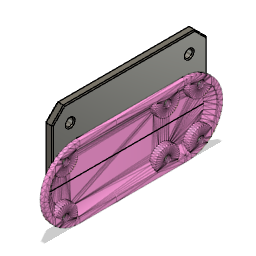
btt-smart-filament-sensor-mount (Autodesk Fusion 360 design; units mm, degrees)
Autodesk Fusion 360 part; units mm, degrees
note: some values were not read from the file. Set by a fixed rule: which sketch regions a step uses.
other "Base Mesh Feature1"
other "Modify1"
sketch "Sketch1" plane through (0, 0, 0) normal (1, 0, 0) x (0, 0, -1)
  line L0 (-32.5, 0) -> (32.5, 0)
  line L1 (32.5, 0) -> (32.5, 24.5)
  line L2 (27.5, 29.5) -> (-27.5, 29.5)
  line L3 (-32.5, 24.5) -> (-32.5, 0)
  line L4 (0, 29.5) -> (0, 0) construction
  circle A0 centre (-25, 22) radius 1.625
  circle A1 centre (25, 22) radius 1.625
  line L5 (27.5, 29.5) -> (32.5, 24.5)
  line L6 (-32.5, 24.5) -> (-27.5, 29.5)
  circle A2 centre (-28.3961, 10.1888) radius 1.5
  circle A3 centre (14.3954, 10.181) radius 1.5
  circle A4 centre (28.3567, 10.1798) radius 1.5
  circle A5 centre (28.3567, 10.1798) radius 3
  circle A6 centre (14.3954, 10.181) radius 3
  circle A7 centre (-28.3961, 10.1888) radius 3
  circle A8 centre (-28.3961, -10.2259) radius 3
  circle A9 centre (14.3954, -10.167) radius 3
  circle A10 centre (28.4406, -10.167) radius 3
  line L7 (22.5, 13) -> (-22.5, 13)
  arc A11 (32.5, 8.2913) -> (22.5, 13) centre (22.5, 0.027) ccw
  line L8 (32.5, 11.1601) -> (31.2931, 9.5653) construction
  arc A12 (-22.5, 13) -> (-32.5, 8.292) centre (-22.5, 0.0257) ccw
  line L9 (-32.5, 11.1715) -> (-31.1644, 9.6829) construction
  line L10 (-31.1644, 9.6829) -> (-32.653, 8.3472) construction
  line L11 (31.2931, 9.5653) -> (32.8879, 8.3584) construction
  point P0 (32.5, 11.1601)
  point P1 (-32.5, 11.1715)
  dimension "d1" = 3.25
  dimension "d2" = 25
  dimension "d3" = 22
  dimension "d4" = 5
  dimension "d5" = 5
  dimension "d6" = 5
  dimension "d7" = 5
  dimension "d8" = 7.5
  dimension "d13" = 3
  dimension "d14" = 3
  dimension "d15" = 3
  dimension "d17" = 6
  dimension "d18" = 6
  dimension "d19" = 6
  dimension "d22" = 6
  dimension "d23" = 6
  dimension "d24" = 6
  dimension "d31" = 7.5
  dimension "d32" = 7.5
  dimension "d33" = 13
  dimension "d34" = 45
  dimension "d35" = 2
  dimension "d36" = 2
  dimension "d37" = 2
  dimension "d38" = 2
  constraint horizontal L0
  constraint vertical L1
  constraint horizontal L2
  constraint vertical L3
  constraint horizontal L4.end L0.start
  constraint coincident L4.end origin
  constraint equal A0 A1
  constraint horizontal A0.centre A1.centre
  constraint symmetric L4 A0.centre A1.centre
  constraint coincident L2 L4.start
  constraint coincident L0 L3.end
  constraint concentric A3 A6
  constraint concentric A2 A7
  constraint vertical A2.centre A8.centre
  constraint vertical A3.centre A9.centre
  constraint horizontal L7
  constraint symmetric L4 L7.start L7.end
  constraint coincident A4.centre A5.centre
  constraint coincident L1 A11.start
  constraint tangent L7 A11
  constraint coincident L1 P0
  constraint coincident P0 L8.start
  constraint coincident A5 L8.end
  constraint coincident A11 L8.end
  constraint coincident L3 P1
  constraint tangent L7 A12
  constraint coincident L3 A12.end
  constraint coincident P1 L9.start
  constraint coincident A12 L9.end
  constraint perpendicular L9 L10
  constraint tangent A12 L10
  constraint perpendicular L8 L11
  measures "d1" diameter of A0
  measures "d2" horizontal distance of L4.end A0.centre
  measures "d3" vertical distance of L4.end A0.centre
  measures "d4" vertical distance of L3.start L2.end
  measures "d5" horizontal distance of L3.start L2.end
  measures "d6" horizontal distance of L2.start L1.end
  measures "d7" vertical distance of L2.start L1.end
  measures "d8" vertical distance of A0.centre L2.end
  measures "d13" diameter of A2
  measures "d14" diameter of A3
  measures "d15" diameter of A4
  measures "d17" diameter of A5
  measures "d18" diameter of A6
  measures "d19" diameter of A7
  measures "d22" diameter of A8
  measures "d23" diameter of A9
  measures "d24" diameter of A10
  measures "d31" horizontal distance of A1.centre L1.end
  measures "d32" horizontal distance of A0.centre L3.start
  measures "d33" vertical distance of L4.end L7.end
  measures "d34" distance of L7.start L7.end
  measures "d35" distance of P0 L8.end
  measures "d36" distance of P1 L9.end
  measures "d37" distance of L9.end L10.end
  measures "d38" distance of L8.end L11.end
extrude "Extrude1" add sketch "Sketch1" along normal blind 3 contours L1 L2 L3 L5 L6 A5 A6 A7 L7 A11 A12 makes body 1
extrude "Extrude2" add sketch "Sketch1" along normal blind 1.9 contours L0 L1 L3 A5 A6 A7 L7 A11 A12 bodies 1
extrude "Extrude5" add sketch "Sketch1" along normal blind 0.2 from surface at 2.88 separate body contours A2 A7 A12 | A2 A7 A12 | A4 A5 A11 | A4 A5 A11 | A2 A12 | A2 A12 | A4 A11 | A4 A11 | A6 L7 | A6 L7 | A3 | A8 | A9 | A10 makes body 2 at (3.08, 9.7459, -27.4557) makes body 3 at (2.88, -11.2657, 27.7532) makes body 4 at (2.88, 11.1119, -14.6113) makes body 5 at (2.88, -11.2068, -29.0834) makes body 6 at (2.88, -9.3188, -13.3319) makes body 7 at (2.88, 11.0325, 28.1933)
chamfer "Chamfer2" distance 0.4 angle 45 10 edges at (3, 16.3956, -32.5) (0, 12.25, -32.5) (0, 27, -30) (3, 27, -30) (3, 29.5, 0) (0, 29.5, 0) (0, 27, 30) (3, 27, 30) (3, 16.396, 32.5) (0, 12.25, 32.5) on bodies 1
chamfer "Chamfer3" distance 0.4 angle 45 7 edges at (0, 22.5876, -23.485) (3, 22.5876, -23.485) (3, 22.5876, 26.515) (0, 22.5876, 26.515) (0, 9.095, -25.5597) (0, 9.0962, -11.5984) (0, 9.1039, 31.193) on bodies 1
